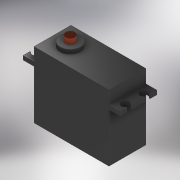
# Autodesk Inventor part: servo_motor
Saved by Autodesk Inventor 2020 (Build 240168000, 168)
## iProperties
Created: 2020-03-24
Part Number: servo_motor
Material: Generic
Document SubType Name: Modeling
Designer: pc-konvi
Density: 1 g/cm^3
Appearance: Glossy - Black
Author: pc-konvi
Autodesk Inventor part; units mm, degrees
ref_plane "XZ Plane" through (0, 0, 0) normal (0, 1, 0) x (-1, 0, 0)
ref_plane "XY Plane" through (0, 0, 0) normal (0, 0, 1) x (1, 0, 0)
sketch "Sketch1" plane through (0, 0, 0) normal (0, 0, 1) x (1, 0, 0)
  line L0 (20.4, -18) -> (-20.4, -18)
  line L1 (-20.4, -18) -> (-20.4, 18)
  line L2 (-20.4, 18) -> (20.4, 18)
  line L3 (20.4, 18) -> (20.4, -18)
  line L4 (20.4, -18) -> (-20.4, 18) construction
  line L5 (-20.4, -18) -> (20.4, 18) construction
  line L6 (-20.4, 8.65) -> (-26.42, 8.65)
  line L7 (-26.42, 8.65) -> (-26.42, 10.7859)
  line L8 (-26.42, 10.7859) -> (-20.4, 10.7859)
  line L9 (-20.4, 10.7859) -> (-20.4, 8.65)
  line L10 (20.4, 10.7859) -> (26.42, 10.7859)
  line L11 (26.42, 10.7859) -> (26.42, 8.65)
  line L12 (26.42, 8.65) -> (20.4, 8.65)
  line L13 (20.4, 8.65) -> (20.4, 10.7859)
  point P0 (0, 0)
  point P1 (20.4, 9.7179)
  point P2 (20.4, 0)
  point P3 (-20.4, 10.7859)
  dimension "d0" = 36
  dimension "d1" = 40.8
  dimension "d2" = 9.35
  dimension "d3" = 9.35
  dimension "d4" = 26.42
  dimension "d5" = 26.42
  constraints: 28 end point, 6 parallel, 4 midpoint, 3 horizontal, 3 perpendicular, 1 point on line, 1 vertical alignment
  measures "d0" distance of L0.end L1.end
  measures "d1" distance of L1.end L2.end
  measures "d2" distance between parallel lines of L2 L12
  measures "d3" distance between parallel lines of L2 L6
  measures "d4" distance from line of point (0, 0) L7
  measures "d5" distance from line of point (0, 0) L11
extrude "Extrusion1" add sketch "Sketch1" along normal blind 10.05
sketch "Sketch2" plane through (-20.4, 18, 0) normal (0, 1, 0) x (1, 0, 0)
  line L0 (40.8, 0) -> (0, 0) projected
  circle A0 centre (9.66, 0) radius 2.5
  circle A1 centre (-3.81, -5.025) radius 2.19
  line L1 (0, 0) -> (0, -10.05) projected
  line L2 (40.8, 0) -> (40.8, -10.05) projected
  line L3 (40.8, 0) -> (39.88, 0)
  line L4 (39.88, 0) -> (39.88, -9.91)
  line L5 (39.88, -9.91) -> (40.8, -9.91)
  line L6 (40.8, -9.91) -> (40.8, 0)
  circle A2 centre (44.61, -5.025) radius 2.19
  line L7 (46.82, 0) -> (40.8, 0) projected
  line L8 (46.82, 0) -> (46.82, -10.05) projected
  line L9 (40.8, 0) -> (46.82, 0)
  line L10 (46.82, 0) -> (46.82, -0.5)
  line L11 (46.82, -0.5) -> (40.8, -0.5)
  line L12 (40.8, -0.5) -> (40.8, 0)
  line L13 (44.3677, -6.275) -> (48.2681, -6.275)
  line L14 (48.2681, -6.275) -> (48.2681, -3.775)
  line L15 (48.2681, -3.775) -> (44.3677, -3.775)
  line L16 (44.3677, -3.775) -> (44.3677, -6.275)
  line L17 (-8.2865, -6.275) -> (-4.5719, -6.275)
  line L18 (-4.5719, -6.275) -> (-4.5719, -3.775)
  line L19 (-4.5719, -3.775) -> (-8.2865, -3.775)
  line L20 (-8.2865, -3.775) -> (-8.2865, -6.275)
  circle A3 centre (9.66, 0) radius 5.5
  line L21 (0, -10.05) -> (-6.02, -10.05) projected
  point P0 (20.4, 0)
  point P1 (0, -5.025)
  point P2 (-4.5719, -5.025)
  point P3 (44.3677, -5.025)
  point P4 (46.4082, -3.775)
  point P5 (46.4082, -6.275)
  point P6 (-5.6082, -6.275)
  point P7 (-5.6082, -3.775)
  point P8 (4.16, 0)
  point P9 (15.16, 0)
  point P10 (12.16, 0)
  point P11 (7.16, 0)
  dimension "d8" = 5
  dimension "d9" = 4.38
  dimension "d10" = 13.47
  dimension "d11" = 9.66
  dimension "d12" = 30.22
  dimension "d13" = 4.38
  dimension "d15" = 0.5
  dimension "d16" = 2.5
  dimension "d17" = 2.5
  dimension "d20" = 3
  dimension "d25" = 3.81
  dimension "d27" = 5.025
  dimension "d28" = 3.81
  dimension "d29" = 10.74
  constraints: 32 end point, 8 parallel, 4 centre point, 4 horizontal, 4 horizontal alignment, 4 perpendicular, 3 midpoint, 2 point on line
  measures "d8" diameter of A0
  measures "d9" diameter of A1
  measures "d10" horizontal distance of A0.centre A1.centre
  measures "d11" distance from line of L1 A0.centre
  measures "d12" distance from line of L4 A0.centre
  measures "d13" diameter of A2
  measures "d15" distance between parallel lines of L11 L7
  measures "d16" distance of L19.end L17.start
  measures "d17" distance of L13.end L14.end
  measures "d20" radial gap between concentric circles of A0 A3
  measures "d25" distance from line of L1 A1.centre
  measures "d27" distance from line of L21 A1.centre
  measures "d28" distance from line of L6 A2.centre
  measures "d29" distance of point (20.4, 0) A0.centre
extrude "Extrusion2" cut sketch "Sketch2" against normal blind 9.91 contours L15 L14 L13 L8 | L8 L13 A2 L15 | L15 L16 L13 A2 | A2 L13 L16 L15 | A1 L17 L18 L19 | L19 L18 L17 A1 | A1 L17 L20 L19
extrude "Extrusion3" add sketch "Sketch2" along normal blind 2.33 contours A3 L0 A0 picked at (14.0825, -0.6382)
extrude "Extrusion4" add sketch "Sketch2" along normal blind 5.38 contours A0 L0 | L0 A0
mirror "Mirror1" about plane through (0, 0, 0) normal (0, 0, 1) of "Extrusion1", "Extrusion2", "Extrusion3"
ref_plane "Work Plane1" through (-10.74, 0, 0) normal (1, 0, 0) x (0, 1, 0)
equation "\"d3\" = d2"
equation "\"d5\" = d4"
equation "\"d13\" = d9"
equation "\"d17\" = d16"
equation "\"d28\" = d25"
body "Solid1"
